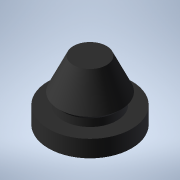
# Autodesk Inventor part: 0000-00186369(1)
Saved by Autodesk Inventor 2021 (Build 250183000, 183)
## iProperties
Created: 2025-07-29
Part Number: 0000-00186369(1)
Material: Generic
Catalog Web Link: www.cadenas.de
Description: Hinge Plug AX 2.0-Hinge Plug AX 2.0
Vendor: RITTAL
Document SubType Name: Modeling
Designer: psAdmin
Manufacturer: RITTAL
Mass: 0.309162 g
Surface Area: 3.09058 cm^2
Volume: 0.309162 cm^3
Density: 1 g/cm^3
Appearance: PSOLRGB-176-176-176
Category: PARTsolutions
Company: RITTAL
Title: 0000-00186369(1)
Author: Cadenas PARTsolutions
Comments: Hinge Plug AX 2.0
PSOL_IDENT_0: {$CADENAS_DATA/23d-libs/rittal/schaltschranksys/kompakt_schaltschr/parts_ae_2_0/hinge_plug_ax_2_0.pr
PSOL_IDENT_1: j},195 {VTYP=3D},{NB=0000-00186369(1)},{LINA=0000-00186369(1)},{NN=Hinge Plug AX 2.0},{DATE=27.11.20
PSOL_IDENT_2: 19 12:11:29},{GEOMDATE=04.09.2019 10:19:13},{VERSION=},{LINEID=10},{WBVAR=DETAIL},{WBNUMERIC=DETAIL}
PSOL_IDENT_3: {NB=0000-00186369(1)},{LINA=0000-00186369(1)},{KT=DUMMY},{BEST=0000-00186369},{DETAIL=1}
NB: 0000-00186369(1)
NN: Hinge Plug AX 2.0
NT: Hinge Plug AX 2.0
NBSYN: $BEST.($DETAIL.)
LINA: 0000-00186369(1)
CATALOG: Rittal
BEST: 0000-00186369
DETAIL: hoch
SUPPLIER: RITTAL
ARTICLENO: 0000-00186369(1)
BOMINFO: 0000-00186369(1)
CREATOR: CADENAS GmbH
Autodesk Inventor part; units mm, degrees
sketch "Sketch_1" plane through (0, 0, 0) normal (0, 0, 1) x (1, 0, 0)
  line L0 (0, -2.029) -> (0, 5.16)
  line L1 (0, 5.16) -> (2, 5.16)
  line L2 (2, 5.16) -> (3.7491, 1.4091)
  line L3 (3.7491, 1.4091) -> (3.25, 0.91)
  line L4 (3.25, 0.91) -> (3.25, 0)
  line L5 (3.25, 0) -> (5, 0)
  line L6 (5, 0) -> (5, -2.029)
  line L7 (5, -2.029) -> (0, -2.029)
  line L8 (0, -2.029) -> (0, 5.16)
  constraints: 18 end point
revolve "Revolution1" add sketch "Sketch_1" angle 360 about axis through (0, -2.029, 0) along (0, -1, 0)
ref_plane "Hinge_Plug_XY" through (0, 0, 0) normal (0, 1, 0) x (1, 0, 0)
ref_plane "Hinge_Plug_YZ" through (0, 0, 0) normal (1, 0, 0) x (0, 0, -1)
ref_plane "Hinge_Plug_ZX" through (0, 0, 0) normal (0, 0, -1) x (0, 1, 0)
body "Solid1"
